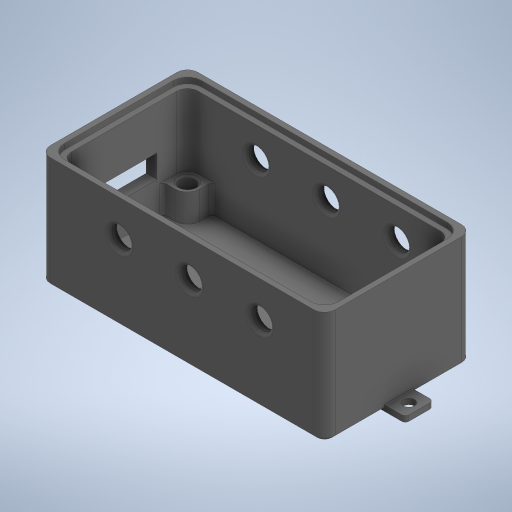
# Autodesk Inventor part: current_sensor_base
Saved by Autodesk Inventor 2023 (Build 270158000, 158)
## iProperties
Created: 2023-10-27
Part Number: current_sensor_base
Material: Generic
Document SubType Name: Modeling
Designer: mark
Density: 1 g/cm^3
Appearance: Default
Author: mark
Autodesk Inventor part; units mm, degrees
ref_plane "YZ Plane" through (0, 0, 0) normal (1, 0, 0) x (0, 1, 0)
ref_plane "XZ Plane" through (0, 0, 0) normal (0, 1, 0) x (-1, 0, 0)
ref_plane "XY Plane" through (0, 0, 0) normal (0, 0, 1) x (1, 0, 0)
sketch "Sketch1" plane through (0, 0, 0) normal (0, 1, 0) x (-1, 0, 0)
  line L0 (34.5, -18) -> (-34.5, -18)
  line L1 (-37.5, -15) -> (-37.5, 15)
  line L2 (-34.5, 18) -> (34.5, 18)
  line L3 (37.5, 15) -> (37.5, -15)
  line L4 (37.5, -21) -> (-37.5, -21)
  line L5 (-40.5, -18) -> (-40.5, 18)
  line L6 (-37.5, 21) -> (37.5, 21)
  line L7 (40.5, 18) -> (40.5, -18)
  arc A0 (37.5, -21) -> (40.5, -18) centre (37.5, -18) ccw
  arc A1 (34.5, -18) -> (37.5, -15) centre (34.5, -15) ccw
  arc A2 (40.5, 18) -> (37.5, 21) centre (37.5, 18) ccw
  arc A3 (37.5, 15) -> (34.5, 18) centre (34.5, 15) ccw
  arc A4 (-34.5, 18) -> (-37.5, 15) centre (-34.5, 15) ccw
  arc A5 (-37.5, 21) -> (-40.5, 18) centre (-37.5, 18) ccw
  arc A6 (-40.5, -18) -> (-37.5, -21) centre (-37.5, -18) ccw
  arc A7 (-37.5, -15) -> (-34.5, -18) centre (-34.5, -15) ccw
  point P0 (0, 0)
  point P1 (-37.5, -18)
  point P2 (37.5, 18)
  point P3 (37.5, 0)
  point P4 (40.5, 0)
  dimension "d0" = 75
  dimension "d1" = 36
  dimension "d2" = 3
  dimension "d3" = 3
  dimension "d4" = 3
  dimension "d5" = 3
  dimension "d6" = 3
  dimension "d23" = 18
  dimension "d24" = 37.5
  constraints: 16 end point, 16 point on circle, 16 tangent, 8 centre point, 7 equal radius, 6 point on line, 4 parallel, 2 horizontal, 2 midpoint, 2 perpendicular
  measures "d0" distance of point (37.5, -18) point (-37.5, -18)
  measures "d1" distance of point (37.5, 18) point (37.5, -18)
  measures "d2" distance between parallel lines of L0 L4
  measures "d3" distance of point (37.5, 0) point (40.5, 0)
  measures "d4" distance between parallel lines of L6 L2
  measures "d5" distance between parallel lines of L5 L1
  measures "d6" radius of A0
  measures "d23" distance from line of point (0, 0) L0
  measures "d24" distance from line of point (0, 0) L3
extrude "Extrusion1" add sketch "Sketch1" along normal blind 30
extrude "Extrusion2" add sketch "Sketch1" against normal blind 2 contours L0 A7 L1 A4 L2 A3 L3 A1 | L4 A6 L5 A5 L6 A2 L7 A0
sketch "Sketch2" plane through (0, 0, 0) normal (0, 1, 0) x (1, 0, 0)
  circle A0 centre (-34, 14.5) radius 2.25
  line L0 (-37.5, -15) -> (-37.5, 15) projected
  line L1 (-34.5, 18) -> (34.5, 18) projected
  line L2 (-37.5, 18) -> (-30.5, 18)
  line L3 (-37.5, 11) -> (-37.5, 18)
  line L4 (-37.5, 11) -> (-30.5, 11)
  line L5 (-30.5, 11) -> (-30.5, 18)
  circle A1 centre (34, 14.5) radius 2.25
  line L6 (37.5, 11) -> (37.5, 18)
  line L7 (30.5, 11) -> (37.5, 11)
  line L8 (30.5, 11) -> (30.5, 18)
  line L9 (30.5, 18) -> (37.5, 18)
  circle A2 centre (-34, -14.5) radius 2.25
  line L10 (-30.5, -18) -> (-30.5, -11)
  line L11 (-37.5, -18) -> (-30.5, -18)
  line L12 (-37.5, -18) -> (-37.5, -11)
  line L13 (-37.5, -11) -> (-30.5, -11)
  circle A3 centre (34, -14.5) radius 2.25
  line L14 (37.5, -18) -> (37.5, -11)
  line L15 (30.5, -18) -> (37.5, -18)
  line L16 (30.5, -18) -> (30.5, -11)
  line L17 (30.5, -11) -> (37.5, -11)
  point P0 (0, 0)
  dimension "d11" = 4.5
  dimension "d12" = 3.5
  dimension "d13" = 3.5
  dimension "d14" = 7
  dimension "d15" = 7
  dimension "d27" = 68
  dimension "d30" = 29
  constraints: 32 end point, 4 centre point, 3 horizontal, 2 collinear, 1 perpendicular, 1 vertical, 30 other
  measures "d11" diameter of A0
  measures "d12" distance from line of L0 A0.centre
  measures "d13" distance from line of L1 A0.centre
  measures "d14" distance of L4.end L3.start
  measures "d15" distance of L2.end L4.end
  measures "d27" distance of A0.centre A1.centre
  measures "d30" distance of A0.centre A2.centre
extrude "Extrusion3" add sketch "Sketch2" along normal blind 8
chamfer "Chamfer1" distance 0.5 angle 45 4 edges at (-36.25, 8, -14.5) (31.75, 8, -14.5) (31.75, 8, 14.5) (-36.25, 8, 14.5)
fillet "Fillet2" radius 3.5 4 edges at (-30.5, 4, -11) (-30.5, 4, 11) (30.5, 4, -11) (30.5, 4, 11)
fillet "Fillet2" radius 1 8 edges at (37.5, 4, -11) (30.5, 4, -18) (-37.5, 4, -11) (-30.5, 4, -18) (-30.5, 4, 18) (-37.5, 4, 11) (30.5, 4, 18) (37.5, 4, 11)
sketch "Sketch3" plane through (-40.5, 30, -18) normal (-1, 0, 0) x (0, 0, 1)
  line L0 (8.75, -20.5) -> (27.25, -20.5)
  line L1 (27.25, -20.5) -> (27.25, -14)
  line L2 (27.25, -14) -> (8.75, -14)
  line L3 (8.75, -14) -> (8.75, -20.5)
  line L4 (-3, -32) -> (-3, 0) projected
  line L5 (8, -22) -> (3, -22) projected
  point P0 (18, -30)
  dimension "d35" = 18.5
  dimension "d36" = 6.5
  dimension "d37" = 11.75
  dimension "d38" = 1.5
  constraints: 8 end point, 2 parallel, 1 horizontal, 1 perpendicular
  measures "d35" distance of L2.end L1.end
  measures "d36" distance of L1.end L0.end
  measures "d37" distance between parallel lines of L4 L3
  measures "d38" distance between parallel lines of L0 L5
extrude "Extrusion4" cut sketch "Sketch3" against normal blind 8
sketch "Sketch4" plane through (0, 30, 0) normal (0, 1, 0) x (1, 0, 0)
  line L0 (-35, 19.5) -> (35, 19.5)
  line L1 (39, 15.5) -> (39, -15.5)
  line L2 (35, -19.5) -> (-35, -19.5)
  line L3 (-39, -15.5) -> (-39, 15.5)
  line L4 (-34.5, 18) -> (34.5, 18) projected
  line L5 (-37.5, -15) -> (-37.5, 15) projected
  line L6 (34.5, -18) -> (-34.5, -18) projected
  line L7 (37.5, 15) -> (37.5, -15) projected
  arc A0 (39, 15.5) -> (35, 19.5) centre (35, 15.5) ccw
  arc A1 (35, -19.5) -> (39, -15.5) centre (35, -15.5) ccw
  arc A2 (-39, -15.5) -> (-35, -19.5) centre (-35, -15.5) ccw
  arc A3 (-35, 19.5) -> (-39, 15.5) centre (-35, 15.5) ccw
  point P0 (0, 0)
  point P1 (-39, 0)
  dimension "d41" = 1.5
  dimension "d42" = 1.5
  dimension "d43" = 1.5
  dimension "d44" = 1.5
  dimension "d45" = 4
  constraints: 8 end point, 8 point on circle, 8 tangent, 4 centre point, 3 equal radius, 2 parallel, 1 horizontal, 1 midpoint, 1 perpendicular
  measures "d41" distance between parallel lines of L4 L0
  measures "d42" distance from line of L5 point (-39, 0)
  measures "d43" distance between parallel lines of L2 L6
  measures "d44" distance between parallel lines of L7 L1
  measures "d45" radius of A0
extrude "Extrusion5" cut sketch "Sketch4" against normal blind 1.6
chamfer "Chamfer2" distance 1 angle 45 8 edges at (0, -2, 21) (-39.6213, -2, 20.1213) (-40.5, -2, 0) (-39.6213, -2, -20.1213) (0, -2, -21) (39.6213, -2, -20.1213) (40.5, -2, 0) (39.6213, -2, 20.1213)
sketch "Sketch6" plane through (-37.5, 30, 21) normal (0, 0, 1) x (1, 0, 0)
  line L0 (0, 0) -> (75, 0) projected
  line L1 (-3, -31) -> (-3, 0) projected
  point P0 (37.5, -30)
  point P1 (19.5, -10.37)
  dimension "d51" = 10.37
  dimension "d52" = 22.5
  measures "d51" distance from line of L0 point (19.5, -10.37)
  measures "d52" distance from line of L1 point (19.5, -10.37)
hole "Hole1" at (-18, 19.63, 21) direction (0, 0, -1) diameter 6 end through all
fillet "Fillet3" radius 1 4 edges at (-18, 22.63, 21) (-18, 22.63, -21) (-18, 22.63, -18) (-18, 22.63, 18)
pattern_linear "Rectangular Pattern1" count 3 spacing 20 along (1, 0, 0) of "Hole1", "Fillet3"
sketch "Sketch7" plane through (0, -2, 0) normal (0, -1, 0) x (1, 0, 0)
  line L0 (45.5, -4) -> (-45.5, -4)
  line L1 (-46.5, -3) -> (-46.5, 3)
  line L2 (-45.5, 4) -> (45.5, 4)
  line L3 (46.5, 3) -> (46.5, -3)
  line L4 (40.5, -18) -> (40.5, 18) projected
  line L5 (-40.5, 18) -> (-40.5, -18) projected
  circle A0 centre (43.5, 0) radius 1.6
  arc A1 (45.5, -4) -> (46.5, -3) centre (45.5, -3) ccw
  arc A2 (46.5, 3) -> (45.5, 4) centre (45.5, 3) ccw
  arc A3 (-46.5, -3) -> (-45.5, -4) centre (-45.5, -3) ccw
  arc A4 (-45.5, 4) -> (-46.5, 3) centre (-45.5, 3) ccw
  circle A5 centre (-43.5, 0) radius 1.6
  point P0 (0, 0)
  dimension "d64" = 6
  dimension "d65" = 6
  dimension "d66" = 8
  dimension "d67" = 4
  dimension "d68" = 3.2
  dimension "d69" = 3
  dimension "d70" = 1
  dimension "d71" = 3.2
  dimension "d72" = 3
  constraints: 8 end point, 8 point on circle, 8 tangent, 6 centre point, 3 equal radius, 2 parallel, 1 horizontal, 1 perpendicular
  measures "d64" distance between parallel lines of L4 L3
  measures "d65" distance between parallel lines of L5 L1
  measures "d66" distance between parallel lines of L2 L0
  measures "d67" distance from line of point (0, 0) L0
  measures "d68" diameter of A0
  measures "d69" distance from line of L3 A0.centre
  measures "d70" radius of A1
  measures "d71" diameter of A5
  measures "d72" distance from line of L1 A5.centre
extrude "Extrusion6" add sketch "Sketch7" against normal blind 1.6
equation "\"d3\" = d2"
equation "\"d4\" = d2"
equation "\"d5\" = d2"
equation "\"d13\" = d12"
equation "\"d42\" = d41"
equation "\"d43\" = d41"
equation "\"d44\" = d41"
equation "\"d65\" = d64"
equation "\"d67\" = 0.5 * d66"
equation "\"d69\" = 0.5 * d64"
equation "\"d71\" = d68"
equation "\"d72\" = d69"
body "Solid1"
